Autodesk Inventor part; units mm, degrees
(part 2 of 3)
sketch "스케치16" plane through (0, 0, 0) normal (0, 0, -1) x (-1, 0, 0)
  line L0 (6.921, -57.5) -> (6.921, -59.5) projected
  arc A0 (4.7026, -59.56) -> (6.921, -59.5) centre (5.811, -59.5) ccw projected
  line L1 (4.7026, -59.56) -> (-3.9306, -59.56) projected
  arc A1 (-6.149, -59.5) -> (-3.9306, -59.56) centre (-5.039, -59.5) ccw projected
  line L2 (-6.149, -59.5) -> (-6.149, -57.5) projected
  arc A2 (-3.9306, -57.44) -> (-6.149, -57.5) centre (-5.039, -57.5) ccw projected
  line L3 (-3.9306, -57.44) -> (4.7026, -57.44) projected
  arc A3 (6.921, -57.5) -> (4.7026, -57.44) centre (5.811, -57.5) ccw projected
  line L4 (-14.6916, -62.5) -> (14.3356, -62.5) projected
  arc A4 (14.3356, -62.5) -> (14.361, -62.05) centre (10.361, -62.05) ccw projected
  line L5 (14.361, -62.05) -> (14.361, -54.5339) projected
  arc A5 (14.361, -54.5339) -> (14.2456, -53.5801) centre (10.361, -54.5339) ccw projected
  line L6 (14.2456, -53.5801) -> (5.6489, -18.5692) projected
  arc A6 (5.6489, -18.5692) -> (-6.0049, -18.5692) centre (-0.178, -20) ccw projected
  line L7 (-6.0049, -18.5692) -> (-14.6016, -53.5801) projected
  arc A7 (-14.6016, -53.5801) -> (-14.717, -54.5339) centre (-10.717, -54.5339) ccw projected
  line L8 (-14.717, -54.5339) -> (-14.717, -62.05) projected
  arc A8 (-14.717, -62.05) -> (-14.6916, -62.5) centre (-10.717, -62.05) ccw projected
  circle A9 centre (10.361, -60) radius 1.35 projected
  line L9 (-8.8997, -47.1327) -> (-4.8208, -30.5211) projected
  arc A10 (-0.6725, -27.4837) -> (-4.8208, -30.5211) centre (-0.9362, -31.475) ccw projected
  arc A11 (-0.6725, -27.4837) -> (0.3165, -27.4837) centre (-0.178, -20) ccw projected
  arc A12 (4.4648, -30.5211) -> (0.3165, -27.4837) centre (0.5802, -31.475) ccw projected
  line L10 (4.4648, -30.5211) -> (8.5437, -47.1327) projected
  arc A13 (5.3379, -52.0285) -> (8.5437, -47.1327) centre (4.6591, -48.0865) ccw projected
  arc A14 (-5.694, -52.0285) -> (5.3379, -52.0285) centre (-0.178, -20) ccw projected
  arc A15 (-8.8997, -47.1327) -> (-5.694, -52.0285) centre (-5.0151, -48.0865) ccw projected
  circle A16 centre (-10.639, -60) radius 1.35 projected
  circle A17 centre (-0.178, -20) radius 4 projected
  line L11 (-16.116, -62.5) -> (15.916, -62.5) projected
  arc A18 (15.916, -62.5) -> (16.439, -60.05) centre (10.439, -60.05) ccw projected
  line L12 (16.439, -60.05) -> (16.439, -54.5339) projected
  arc A19 (16.439, -54.5339) -> (16.2659, -53.1031) centre (10.439, -54.5339) ccw projected
  line L13 (16.2659, -53.1031) -> (7.6692, -18.0923) projected
  arc A20 (7.6692, -18.0923) -> (-7.8692, -18.0923) centre (-0.1, -20) ccw projected
  line L14 (-7.8692, -18.0923) -> (-16.4659, -53.1031) projected
  arc A21 (-16.4659, -53.1031) -> (-16.639, -54.5339) centre (-10.639, -54.5339) ccw projected
  line L15 (-16.639, -54.5339) -> (-16.639, -60.05) projected
  arc A22 (-16.639, -60.05) -> (-16.116, -62.5) centre (-10.639, -60.05) ccw projected
  arc A23 (-6.149, -59.5) -> (-3.9306, -59.56) centre (-5.039, -59.5) ccw projected
  line L16 (-6.149, -59.5) -> (-6.149, -57.5) projected
  arc A24 (-3.9306, -57.44) -> (-6.149, -57.5) centre (-5.039, -57.5) ccw projected
  line L17 (-3.9306, -57.44) -> (4.7026, -57.44) projected
  arc A25 (6.921, -57.5) -> (4.7026, -57.44) centre (5.811, -57.5) ccw projected
  line L18 (6.921, -57.5) -> (6.921, -59.5) projected
  arc A26 (4.7026, -59.56) -> (6.921, -59.5) centre (5.811, -59.5) ccw projected
  line L19 (4.7026, -59.56) -> (-3.9306, -59.56) projected
  line L20 (-8.16, -47.3) -> (-8.16, -43.3) projected
  arc A27 (-4.0409, -43.24) -> (-8.16, -43.3) centre (-6.1, -43.3) ccw projected
  line L21 (-4.0409, -43.24) -> (3.8409, -43.24) projected
  arc A28 (7.96, -43.3) -> (3.8409, -43.24) centre (5.9, -43.3) ccw projected
  line L22 (7.96, -43.3) -> (7.96, -47.3) projected
  arc A29 (3.8409, -47.36) -> (7.96, -47.3) centre (5.9, -47.3) ccw projected
  line L23 (3.8409, -47.36) -> (-4.0409, -47.36) projected
  arc A30 (-8.16, -47.3) -> (-4.0409, -47.36) centre (-6.1, -47.3) ccw projected
  line L24 (5.1861, -28.9475) -> (7.0991, -36.7384) projected
  arc A31 (5.7409, -39.1281) -> (7.0991, -36.7384) centre (5.1568, -37.2153) ccw projected
  arc A32 (-5.9409, -39.1281) -> (5.7409, -39.1281) centre (-0.1, -20) ccw projected
  arc A33 (-7.2991, -36.7384) -> (-5.9409, -39.1281) centre (-5.3568, -37.2153) ccw projected
  line L25 (-7.2991, -36.7384) -> (-5.3861, -28.9475) projected
  arc A34 (-2.775, -27.5395) -> (-5.3861, -28.9475) centre (-3.4438, -29.4244) ccw projected
  arc A35 (-2.775, -27.5395) -> (2.575, -27.5395) centre (-0.1, -20) ccw projected
  arc A36 (5.1861, -28.9475) -> (2.575, -27.5395) centre (3.2438, -29.4244) ccw projected
  circle A37 centre (-11.1, -45.3) radius 1.35 projected
  circle A38 centre (10.9, -45.3) radius 1.35 projected
  circle A39 centre (-0.1, -20) radius 4 projected
  circle A40 centre (-10.639, -60) radius 1.35 projected
  circle A41 centre (10.361, -60) radius 1.35 projected
  line L26 (-15.5728, -53.3416) -> (-6.9761, -18.3308)
  arc A42 (6.62, -18.3308) -> (-6.9761, -18.3308) centre (-0.178, -20) ccw
  line L27 (6.62, -18.3308) -> (15.2167, -53.3416)
  arc A43 (15.361, -54.5339) -> (15.2167, -53.3416) centre (10.361, -54.5339) ccw
  line L28 (15.361, -54.5339) -> (15.361, -62.05)
  arc A44 (15.1461, -63.5) -> (15.361, -62.05) centre (10.361, -62.05) ccw
  line L29 (15.1461, -63.5) -> (-15.5022, -63.5)
  arc A45 (-15.717, -62.05) -> (-15.5022, -63.5) centre (-10.717, -62.05) ccw
  line L30 (-15.717, -62.05) -> (-15.717, -54.5339)
  arc A46 (-15.5728, -53.3416) -> (-15.717, -54.5339) centre (-10.717, -54.5339) ccw
  point P0 (0, 0)
  point P1 (-15.6967, -62.5)
  point P2 (15.3407, -62.5)
  dimension "d62" = 1
  constraints: 10 end point, 10 point on circle, 5 centre point, 9 other
  measures "d62" distance between parallel lines of L7 L26
extrude "돌출16" cut sketch "스케치16" against normal through all contours L11 A22 L15 A21 L14 A20 L13 A19 L12 A18 A44 L28 A43 L27 A42 L26 A46 L30 A45
sketch "스케치17" plane through (0, 0, 0) normal (0, 0, -1) x (-1, 0, 0)
  circle A0 centre (10.361, -60) radius 1.35 projected
  circle A1 centre (-10.639, -60) radius 1.35 projected
  circle A2 centre (-0.1, -20) radius 4 projected
  circle A3 centre (10.9, -45.3) radius 1.35 projected
  circle A4 centre (-11.1, -45.3) radius 1.35 projected
  line L0 (5.1861, -28.9475) -> (7.0991, -36.7384) projected
  arc A5 (5.7409, -39.1281) -> (7.0991, -36.7384) centre (5.1568, -37.2153) ccw projected
  arc A6 (-5.9409, -39.1281) -> (5.7409, -39.1281) centre (-0.1, -20) ccw projected
  arc A7 (-7.2991, -36.7384) -> (-5.9409, -39.1281) centre (-5.3568, -37.2153) ccw projected
  line L1 (-7.2991, -36.7384) -> (-5.3861, -28.9475) projected
  arc A8 (-2.775, -27.5395) -> (-5.3861, -28.9475) centre (-3.4438, -29.4244) ccw projected
  arc A9 (-2.775, -27.5395) -> (2.575, -27.5395) centre (-0.1, -20) ccw projected
  arc A10 (5.1861, -28.9475) -> (2.575, -27.5395) centre (3.2438, -29.4244) ccw projected
  line L2 (-8.16, -47.3) -> (-8.16, -43.3) projected
  arc A11 (-4.0409, -43.24) -> (-8.16, -43.3) centre (-6.1, -43.3) ccw projected
  line L3 (-4.0409, -43.24) -> (3.8409, -43.24) projected
  arc A12 (7.96, -43.3) -> (3.8409, -43.24) centre (5.9, -43.3) ccw projected
  line L4 (7.96, -43.3) -> (7.96, -47.3) projected
  arc A13 (3.8409, -47.36) -> (7.96, -47.3) centre (5.9, -47.3) ccw projected
  line L5 (3.8409, -47.36) -> (-4.0409, -47.36) projected
  arc A14 (-8.16, -47.3) -> (-4.0409, -47.36) centre (-6.1, -47.3) ccw projected
  arc A15 (-6.149, -59.5) -> (-3.9306, -59.56) centre (-5.039, -59.5) ccw projected
  line L6 (-6.149, -59.5) -> (-6.149, -57.5) projected
  arc A16 (-3.9306, -57.44) -> (-6.149, -57.5) centre (-5.039, -57.5) ccw projected
  line L7 (-3.9306, -57.44) -> (4.7026, -57.44) projected
  arc A17 (6.921, -57.5) -> (4.7026, -57.44) centre (5.811, -57.5) ccw projected
  line L8 (6.921, -57.5) -> (6.921, -59.5) projected
  arc A18 (4.7026, -59.56) -> (6.921, -59.5) centre (5.811, -59.5) ccw projected
  line L9 (4.7026, -59.56) -> (-3.9306, -59.56) projected
  arc A19 (15.3407, -62.5) -> (15.361, -62.05) centre (10.361, -62.05) ccw projected
  line L10 (15.361, -62.05) -> (15.361, -54.5339) projected
  arc A20 (15.361, -54.5339) -> (15.2167, -53.3416) centre (10.361, -54.5339) ccw projected
  line L11 (15.2167, -53.3416) -> (6.62, -18.3308) projected
  arc A21 (6.62, -18.3308) -> (-6.9761, -18.3308) centre (-0.178, -20) ccw projected
  line L12 (-6.9761, -18.3308) -> (-15.5728, -53.3416) projected
  arc A22 (-15.5728, -53.3416) -> (-15.717, -54.5339) centre (-10.717, -54.5339) ccw projected
  line L13 (-15.717, -54.5339) -> (-15.717, -62.05) projected
  arc A23 (-15.717, -62.05) -> (-15.6967, -62.5) centre (-10.717, -62.05) ccw projected
  line L14 (-15.6967, -62.5) -> (15.3407, -62.5) projected
  line L15 (15.361, -54.5339) -> (-15.717, -54.5339)
  line L16 (-15.717, -54.5339) -> (-15.717, -62.5)
  line L17 (-15.717, -62.5) -> (15.361, -62.5)
  line L18 (15.361, -62.5) -> (15.361, -54.5339)
  point P0 (0, 0)
  point P1 (15.361, -62.05)
  point P2 (15.3407, -62.5)
  constraints: 8 end point, 2 parallel, 1 horizontal, 1 perpendicular
extrude "돌출17" add sketch "스케치17" against normal blind 2 contours A19 L18 L17 | L17 L16 A23
sketch "스케치18" plane through (0, 0, 2) normal (0, 0, 1) x (1, 0, 0)
  line L0 (-15.361, -62.5) -> (15.717, -62.5) projected
  line L1 (15.717, -62.5) -> (15.717, -54.5339) projected
  arc A0 (15.717, -54.5339) -> (15.5728, -53.3416) centre (10.717, -54.5339) ccw projected
  line L2 (15.5728, -53.3416) -> (6.9761, -18.3308) projected
  arc A1 (6.9761, -18.3308) -> (-6.62, -18.3308) centre (0.178, -20) ccw projected
  line L3 (-6.62, -18.3308) -> (-15.2167, -53.3416) projected
  arc A2 (-15.2167, -53.3416) -> (-15.361, -54.5339) centre (-10.361, -54.5339) ccw projected
  line L4 (-15.361, -54.5339) -> (-15.361, -62.5) projected
  line L5 (8.16, -43.3) -> (8.16, -47.3) projected
  arc A3 (4.0409, -47.36) -> (8.16, -47.3) centre (6.1, -47.3) ccw projected
  line L6 (4.0409, -47.36) -> (-3.8409, -47.36) projected
  arc A4 (-7.96, -47.3) -> (-3.8409, -47.36) centre (-5.9, -47.3) ccw projected
  line L7 (-7.96, -47.3) -> (-7.96, -43.3) projected
  arc A5 (-3.8409, -43.24) -> (-7.96, -43.3) centre (-5.9, -43.3) ccw projected
  line L8 (-3.8409, -43.24) -> (4.0409, -43.24) projected
  arc A6 (8.16, -43.3) -> (4.0409, -43.24) centre (6.1, -43.3) ccw projected
  line L9 (-7.0991, -36.7384) -> (-5.1861, -28.9475) projected
  arc A7 (-2.575, -27.5395) -> (-5.1861, -28.9475) centre (-3.2438, -29.4244) ccw projected
  arc A8 (-2.575, -27.5395) -> (2.775, -27.5395) centre (0.1, -20) ccw projected
  arc A9 (5.3861, -28.9475) -> (2.775, -27.5395) centre (3.4438, -29.4244) ccw projected
  line L10 (5.3861, -28.9475) -> (7.2991, -36.7384) projected
  arc A10 (5.9409, -39.1281) -> (7.2991, -36.7384) centre (5.3568, -37.2153) ccw projected
  arc A11 (-5.7409, -39.1281) -> (5.9409, -39.1281) centre (0.1, -20) ccw projected
  arc A12 (-7.0991, -36.7384) -> (-5.7409, -39.1281) centre (-5.1568, -37.2153) ccw projected
  circle A13 centre (11.1, -45.3) radius 1.35 projected
  circle A14 centre (-10.9, -45.3) radius 1.35 projected
  circle A15 centre (10.639, -60) radius 1.35 projected
  circle A16 centre (-10.361, -60) radius 1.35 projected
  circle A17 centre (0.1, -20) radius 4 projected
  arc A18 (3.9306, -59.56) -> (6.149, -59.5) centre (5.039, -59.5) ccw projected
  line L11 (3.9306, -59.56) -> (-4.7026, -59.56) projected
  arc A19 (-6.921, -59.5) -> (-4.7026, -59.56) centre (-5.811, -59.5) ccw projected
  line L12 (-6.921, -59.5) -> (-6.921, -57.5) projected
  arc A20 (-4.7026, -57.44) -> (-6.921, -57.5) centre (-5.811, -57.5) ccw projected
  line L13 (-4.7026, -57.44) -> (3.9306, -57.44) projected
  arc A21 (6.149, -57.5) -> (3.9306, -57.44) centre (5.039, -57.5) ccw projected
  line L14 (6.149, -57.5) -> (6.149, -59.5) projected
  point P0 (0, 0)
extrude "돌출18" add sketch "스케치18" against normal blind 2 contours L5 A3 L6 A4 L7 A5 L8 A6 | A13 | A14 | L11 A19 L12 A20 L13 A21 L14 A18
sketch "스케치19" plane through (0, 0, 2) normal (0, 0, 1) x (1, 0, 0)
  line L0 (-15.361, -62.5) -> (15.717, -62.5) projected
  line L1 (15.717, -62.5) -> (15.717, -54.5339) projected
  arc A0 (15.717, -54.5339) -> (15.5728, -53.3416) centre (10.717, -54.5339) ccw projected
  line L2 (15.5728, -53.3416) -> (6.9761, -18.3308) projected
  arc A1 (6.9761, -18.3308) -> (-6.62, -18.3308) centre (0.178, -20) ccw projected
  line L3 (-6.62, -18.3308) -> (-15.2167, -53.3416) projected
  arc A2 (-15.2167, -53.3416) -> (-15.361, -54.5339) centre (-10.361, -54.5339) ccw projected
  line L4 (-15.361, -54.5339) -> (-15.361, -62.5) projected
  line L5 (-7.0991, -36.7384) -> (-5.1861, -28.9475) projected
  arc A3 (-2.575, -27.5395) -> (-5.1861, -28.9475) centre (-3.2438, -29.4244) ccw projected
  arc A4 (-2.575, -27.5395) -> (2.775, -27.5395) centre (0.1, -20) ccw projected
  arc A5 (5.3861, -28.9475) -> (2.775, -27.5395) centre (3.4438, -29.4244) ccw projected
  line L6 (5.3861, -28.9475) -> (7.2991, -36.7384) projected
  arc A6 (5.9409, -39.1281) -> (7.2991, -36.7384) centre (5.3568, -37.2153) ccw projected
  arc A7 (-5.7409, -39.1281) -> (5.9409, -39.1281) centre (0.1, -20) ccw projected
  arc A8 (-7.0991, -36.7384) -> (-5.7409, -39.1281) centre (-5.1568, -37.2153) ccw projected
  circle A9 centre (10.639, -60) radius 1.35 projected
  circle A10 centre (-10.361, -60) radius 1.35 projected
  circle A11 centre (0.1, -20) radius 4 projected
  line L7 (7.199, -57.5) -> (7.199, -59.5) projected
  arc A12 (4.9806, -59.56) -> (7.199, -59.5) centre (6.089, -59.5) ccw projected
  line L8 (4.9806, -59.56) -> (-3.6526, -59.56) projected
  arc A13 (-5.871, -59.5) -> (-3.6526, -59.56) centre (-4.761, -59.5) ccw projected
  line L9 (-5.871, -59.5) -> (-5.871, -57.5) projected
  arc A14 (-3.6526, -57.44) -> (-5.871, -57.5) centre (-4.761, -57.5) ccw projected
  line L10 (-3.6526, -57.44) -> (4.9806, -57.44) projected
  arc A15 (7.199, -57.5) -> (4.9806, -57.44) centre (6.089, -57.5) ccw projected
  line L11 (-14.4136, -62.5) -> (14.6136, -62.5) projected
  arc A16 (14.6136, -62.5) -> (14.639, -62.05) centre (10.639, -62.05) ccw projected
  line L12 (14.639, -62.05) -> (14.639, -54.5339) projected
  arc A17 (14.639, -54.5339) -> (14.5236, -53.5801) centre (10.639, -54.5339) ccw projected
  line L13 (14.5236, -53.5801) -> (5.9269, -18.5692) projected
  arc A18 (5.9269, -18.5692) -> (-5.7269, -18.5692) centre (0.1, -20) ccw projected
  line L14 (-5.7269, -18.5692) -> (-14.3236, -53.5801) projected
  arc A19 (-14.3236, -53.5801) -> (-14.439, -54.5339) centre (-10.439, -54.5339) ccw projected
  line L15 (-14.439, -54.5339) -> (-14.439, -62.05) projected
  arc A20 (-14.439, -62.05) -> (-14.4136, -62.5) centre (-10.439, -62.05) ccw projected
  circle A21 centre (10.639, -60) radius 1.35 projected
  line L16 (-8.6217, -47.1327) -> (-4.5428, -30.5211) projected
  arc A22 (-0.3945, -27.4837) -> (-4.5428, -30.5211) centre (-0.6582, -31.475) ccw projected
  arc A23 (-0.3945, -27.4837) -> (0.5945, -27.4837) centre (0.1, -20) ccw projected
  arc A24 (4.7428, -30.5211) -> (0.5945, -27.4837) centre (0.8582, -31.475) ccw projected
  line L17 (4.7428, -30.5211) -> (8.8217, -47.1327) projected
  arc A25 (5.616, -52.0285) -> (8.8217, -47.1327) centre (4.9371, -48.0865) ccw projected
  arc A26 (-5.416, -52.0285) -> (5.616, -52.0285) centre (0.1, -20) ccw projected
  arc A27 (-8.6217, -47.1327) -> (-5.416, -52.0285) centre (-4.7371, -48.0865) ccw projected
  circle A28 centre (-10.361, -60) radius 1.35 projected
  circle A29 centre (0.1, -20) radius 4 projected
  arc A30 (20.1, 4.5766) -> (19.5808, 6.2636) centre (17.1, 4.5766) ccw projected
  line L18 (19.5808, 6.2636) -> (15.5953, 12.1246) projected
  arc A31 (15.5953, 12.1246) -> (13.9414, 13) centre (13.9414, 11) ccw projected
  line L19 (13, 13) -> (13.9414, 13) projected
  arc A32 (14.5, 11.5) -> (13, 13) centre (13, 11.5) ccw projected
  line L20 (14.5, -41.5) -> (14.5, 11.5) projected
  arc A33 (13.5, -42.5) -> (14.5, -41.5) centre (13.5, -41.5) ccw projected
  line L21 (-13.5, -42.5) -> (13.5, -42.5) projected
  arc A34 (-14.5, -41.5) -> (-13.5, -42.5) centre (-13.5, -41.5) ccw projected
  line L22 (-14.5, 11.5) -> (-14.5, -41.5) projected
  arc A35 (-13, 13) -> (-14.5, 11.5) centre (-13, 11.5) ccw projected
  line L23 (-13.9414, 13) -> (-13, 13) projected
  arc A36 (-13.9414, 13) -> (-15.5953, 12.1246) centre (-13.9414, 11) ccw projected
  line L24 (-15.5953, 12.1246) -> (-19.5808, 6.2636) projected
  arc A37 (-19.5808, 6.2636) -> (-20.1, 4.5766) centre (-17.1, 4.5766) ccw projected
  line L25 (-20.1, 4.5766) -> (-20.1, -39.6766) projected
  arc A38 (-20.1, -39.6766) -> (-19.5808, -41.3636) centre (-17.1, -39.6766) ccw projected
  line L26 (-19.5808, -41.3636) -> (-15.8929, -46.7869) projected
  arc A39 (-15.8929, -46.7869) -> (-13.4121, -48.1) centre (-13.4121, -45.1) ccw projected
  line L27 (-13.4121, -48.1) -> (13.4121, -48.1) projected
  arc A40 (13.4121, -48.1) -> (15.8929, -46.7869) centre (13.4121, -45.1) ccw projected
  line L28 (15.8929, -46.7869) -> (19.5808, -41.3636) projected
  arc A41 (19.5808, -41.3636) -> (20.1, -39.6766) centre (17.1, -39.6766) ccw projected
  line L29 (20.1, -39.6766) -> (20.1, 4.5766) projected
  circle A42 centre (-17.3, 4) radius 1.35 projected
  circle A43 centre (-17.3, -18) radius 1.35 projected
  circle A44 centre (-11, -45.3) radius 1.35 projected
  circle A45 centre (17.3, 4) radius 1.35 projected
  circle A46 centre (17.3, -18) radius 1.35 projected
  circle A47 centre (11, -45.3) radius 1.35 projected
  circle A48 centre (-17.3, -40) radius 1.35 projected
  circle A49 centre (17.3, -40) radius 1.35 projected
  point P0 (0, 0)
extrude "돌출19" cut sketch "스케치19" against normal blind 2 contours A44 L14 | L14 A44 | L7 A12 L8 A13 L9 A14 L10 A15 | A47
sketch "스케치20" plane through (0, 0, 2) normal (0, 0, 1) x (1, 0, 0)
  circle A0 centre (-4.4, -45.3) radius 1 projected
  circle A1 centre (4.4, -45.3) radius 1 projected
  line L0 (8, -43.3) -> (8, -47.3) projected
  line L1 (-8, -43.3) -> (8, -43.3) projected
  line L2 (-8, -47.3) -> (-8, -43.3) projected
  line L3 (8, -47.3) -> (-8, -47.3) projected
  line L4 (-8.06, -47.36) -> (-8.06, -43.24)
  line L5 (-8.06, -43.24) -> (8.06, -43.24)
  line L6 (8.06, -43.24) -> (8.06, -47.36)
  line L7 (8.06, -47.36) -> (-8.06, -47.36)
  line L8 (8.06, -47.36) -> (8.06, -43.24)
  line L9 (-22.2818, -39.9612) -> (-22.2818, -44.0812)
  line L10 (-22.2818, -44.0812) -> (-22.2818, -39.9612) construction
  line L11 (-20.7818, -44.0812) -> (-20.7818, -39.9612)
  line L12 (-23.7818, -39.9612) -> (-23.7818, -44.0812)
  arc A2 (-23.7818, -44.0812) -> (-20.7818, -44.0812) centre (-22.2818, -44.0812) ccw
  arc A3 (-20.7818, -39.9612) -> (-23.7818, -39.9612) centre (-22.2818, -39.9612) ccw
  line L13 (6.56, -43.24) -> (6.56, -47.36)
  line L14 (6.56, -47.36) -> (6.56, -43.24) construction
  line L15 (8.06, -47.36) -> (8.06, -43.24)
  line L16 (5.06, -43.24) -> (5.06, -47.36)
  arc A4 (5.06, -47.36) -> (8.06, -47.36) centre (6.56, -47.36) ccw
  arc A5 (8.06, -43.24) -> (5.06, -43.24) centre (6.56, -43.24) ccw
  line L17 (-6.56, -43.24) -> (-6.56, -47.36)
  line L18 (-6.56, -47.36) -> (-6.56, -43.24) construction
  line L19 (-5.06, -47.36) -> (-5.06, -43.24)
  line L20 (-8.06, -43.24) -> (-8.06, -47.36)
  arc A6 (-8.06, -47.36) -> (-5.06, -47.36) centre (-6.56, -47.36) ccw
  arc A7 (-5.06, -43.24) -> (-8.06, -43.24) centre (-6.56, -43.24) ccw
  point P0 (0, 0)
  point P1 (-22.2818, -42.0212)
  point P2 (6.56, -45.3)
  point P3 (-6.56, -45.3)
  point P4 (5.06, -43.3)
  point P5 (-5.06, -43.3)
  dimension "d71" = 0.06
  dimension "d72" = 3
  dimension "d73" = 3
  dimension "d74" = 3
  constraints: 40 end point, 12 point on circle, 12 tangent, 6 centre point, 4 vertical, 3 midpoint, 3 parallel, 3 other
  measures "d71" distance between parallel lines of L3 L7
  measures "d72" diameter of A3
  measures "d73" diameter of A5
  measures "d74" diameter of A7
extrude "돌출20" cut sketch "스케치20" against normal blind 2 contours A0 L19 | A0 L19 L1 L16 A1 L3 | L19 A0 | A0 L19 L3 L17 L1 | L1 L17 L5 L19 | L19 L7 L17 L3 | L3 L16 L7 L19 | L17 L3 L2 L1 | L1 L2 L3 L17 L7 L4 L5 | L16 L5 L13 L1 | L1 L13 L3 L16 A1 | L5 A7 | L3 L13 L7 L16 | A6 L7 | L13 L5 L6 L7 L3 L0 L1 | L1 L0 L3 L13 | A5 L5 | L16 A1 | A1 L16 | L7 A4
sketch "스케치21" plane through (0, 0, 0) normal (0, 0, -1) x (-1, 0, 0)
  arc A0 (8.06, -43.24) -> (5.06, -43.24) centre (6.56, -43.24) ccw projected
  line L0 (8.06, -43.24) -> (8.06, -47.36) projected
  arc A1 (5.06, -47.36) -> (8.06, -47.36) centre (6.56, -47.36) ccw projected
  line L1 (5.06, -47.36) -> (-5.06, -47.36) projected
  arc A2 (-8.06, -47.36) -> (-5.06, -47.36) centre (-6.56, -47.36) ccw projected
  line L2 (-8.06, -47.36) -> (-8.06, -43.24) projected
  arc A3 (-5.06, -43.24) -> (-8.06, -43.24) centre (-6.56, -43.24) ccw projected
  line L3 (-5.06, -43.24) -> (-5.06, -43.3) projected
  line L4 (-5.06, -43.3) -> (5.06, -43.3) projected
  line L5 (5.06, -43.3) -> (5.06, -43.24) projected
  circle A4 centre (-11, -45.3) radius 1.35 projected
  circle A5 centre (11, -45.3) radius 1.35 projected
  arc A6 (3.6526, -59.56) -> (5.871, -59.5) centre (4.761, -59.5) ccw projected
  line L6 (3.6526, -59.56) -> (-4.9806, -59.56) projected
  arc A7 (-7.199, -59.5) -> (-4.9806, -59.56) centre (-6.089, -59.5) ccw projected
  line L7 (-7.199, -59.5) -> (-7.199, -57.5) projected
  arc A8 (-4.9806, -57.44) -> (-7.199, -57.5) centre (-6.089, -57.5) ccw projected
  line L8 (-4.9806, -57.44) -> (3.6526, -57.44) projected
  arc A9 (5.871, -57.5) -> (3.6526, -57.44) centre (4.761, -57.5) ccw projected
  line L9 (5.871, -57.5) -> (5.871, -59.5) projected
  circle A10 centre (10.361, -60) radius 1.35 projected
  circle A11 centre (-10.639, -60) radius 1.35 projected
  circle A12 centre (-0.1, -20) radius 4 projected
  line L10 (5.1861, -28.9475) -> (7.0991, -36.7384) projected
  arc A13 (5.7409, -39.1281) -> (7.0991, -36.7384) centre (5.1568, -37.2153) ccw projected
  arc A14 (-5.9409, -39.1281) -> (5.7409, -39.1281) centre (-0.1, -20) ccw projected
  arc A15 (-7.2991, -36.7384) -> (-5.9409, -39.1281) centre (-5.3568, -37.2153) ccw projected
  line L11 (-7.2991, -36.7384) -> (-5.3861, -28.9475) projected
  arc A16 (-2.775, -27.5395) -> (-5.3861, -28.9475) centre (-3.4438, -29.4244) ccw projected
  arc A17 (-2.775, -27.5395) -> (2.575, -27.5395) centre (-0.1, -20) ccw projected
  arc A18 (5.1861, -28.9475) -> (2.575, -27.5395) centre (3.2438, -29.4244) ccw projected
  line L12 (15.361, -62.5) -> (15.361, -54.5339) projected
  arc A19 (15.361, -54.5339) -> (15.2167, -53.3416) centre (10.361, -54.5339) ccw projected
  line L13 (15.2167, -53.3416) -> (6.62, -18.3308) projected
  arc A20 (6.62, -18.3308) -> (-6.9761, -18.3308) centre (-0.178, -20) ccw projected
  line L14 (-6.9761, -18.3308) -> (-15.5728, -53.3416) projected
  arc A21 (-15.5728, -53.3416) -> (-15.717, -54.5339) centre (-10.717, -54.5339) ccw projected
  line L15 (-15.717, -54.5339) -> (-15.717, -62.5) projected
  line L16 (-15.717, -62.5) -> (15.361, -62.5) projected
  point P0 (0, 0)
  point P1 (-13.6725, -37.0927)
  constraints: 1 other
extrude "돌출21" add sketch "스케치21" against normal blind 2 contours L0 A1 L1 A2 L2 A3 L3 L4 L5 A0 | A4 | A5 | L6 A7 L7 A8 L8 A9 L9 A6 | A10 | A11
sketch "스케치22" plane through (0, 0, 0) normal (0, 0, -1) x (-1, 0, 0)
  line L0 (7.3148, -57.5317) -> (7.3064, -59.5317) projected
  arc A0 (5.1878, -59.5827) -> (7.3064, -59.5317) centre (6.2464, -59.5272) ccw projected
  line L1 (5.1878, -59.5827) -> (-5.7227, -59.5366) projected
  arc A1 (-7.8407, -59.4676) -> (-5.7227, -59.5366) centre (-6.7807, -59.4721) ccw projected
  line L2 (-7.8407, -59.4676) -> (-7.8323, -57.4676) projected
  arc A2 (-5.7137, -57.4166) -> (-7.8323, -57.4676) centre (-6.7723, -57.4721) ccw projected
  line L3 (-5.7137, -57.4166) -> (5.1968, -57.4628) projected
  arc A3 (7.3148, -57.5317) -> (5.1968, -57.4628) centre (6.2548, -57.5272) ccw projected
  circle A4 centre (-12.2828, -59.9488) radius 1.35 projected
  circle A5 centre (11.7442, -60.0505) radius 1.35 projected
  line L4 (-14.8188, -62.4381) -> (14.259, -62.5612) projected
  line L5 (14.259, -62.5612) -> (14.2927, -54.5951) projected
  arc A6 (14.2927, -54.5951) -> (14.1814, -53.6408) centre (10.2927, -54.5782) ccw projected
  line L6 (14.1814, -53.6408) -> (5.7329, -18.5939) projected
  arc A7 (5.7329, -18.5939) -> (-5.9208, -18.5446) centre (-0.1, -20) ccw projected
  line L7 (-5.9208, -18.5446) -> (-14.6656, -53.5187) projected
  arc A8 (-14.6656, -53.5187) -> (-14.7851, -54.4721) centre (-10.7851, -54.489) ccw projected
  line L8 (-14.7851, -54.4721) -> (-14.8188, -62.4381) projected
  line L9 (-8.9364, -47.0955) -> (-4.7873, -30.5014) projected
  arc A9 (-0.6262, -27.4815) -> (-4.7873, -30.5014) centre (-0.9068, -31.4717) ccw projected
  arc A10 (-0.6262, -27.4815) -> (0.3628, -27.4857) centre (-0.1, -20) ccw projected
  arc A11 (4.4982, -30.5407) -> (0.3628, -27.4857) centre (0.6096, -31.4781) ccw projected
  line L10 (4.4982, -30.5407) -> (8.5068, -47.1694) projected
  arc A12 (5.2803, -52.0515) -> (8.5068, -47.1694) centre (4.6182, -48.1067) ccw projected
  arc A13 (-5.7515, -52.0049) -> (5.2803, -52.0515) centre (-0.1, -20) ccw projected
  arc A14 (-8.9364, -47.0955) -> (-5.7515, -52.0049) centre (-5.0559, -48.0658) ccw projected
  circle A15 centre (-0.1, -20) radius 4 projected
  point P0 (0, 0)
extrude "돌출22" cut sketch "스케치22" against normal blind 2 contours L0 A0 L1 A1 L2 A2 L3 A3 | A4 | A5
sketch "스케치23" plane through (0, 0, 2) normal (0, 0, 1) x (1, 0, 0)
  circle A0 centre (4.607, -45.2811) radius 1 projected
  circle A1 centre (-4.1929, -45.3184) radius 1 projected
  line L0 (-7.8013, -43.3337) -> (-7.7844, -47.3336) projected
  line L1 (8.1985, -43.2659) -> (-7.8013, -43.3337) projected
  line L2 (8.2155, -47.2659) -> (8.1985, -43.2659) projected
  line L3 (-7.7844, -47.3336) -> (8.2155, -47.2659) projected
  circle A2 centre (-10.7928, -45.3463) radius 1 projected
  line L4 (-8.9013, -43.3383) -> (-8.8844, -47.3383) projected
  line L5 (-8.8844, -47.3383) -> (-12.7843, -47.3548) projected
  line L6 (-12.7843, -47.3548) -> (-12.8013, -43.3548) projected
  line L7 (-12.8013, -43.3548) -> (-8.9013, -43.3383) projected
  circle A3 centre (11.207, -45.2532) radius 1 projected
  line L8 (9.3155, -47.2612) -> (9.2985, -43.2613) projected
  line L9 (9.2985, -43.2613) -> (13.1985, -43.2448) projected
  line L10 (13.1985, -43.2448) -> (13.2154, -47.2447) projected
  line L11 (13.2154, -47.2447) -> (9.3155, -47.2612) projected
  circle A4 centre (11.207, -45.2532) radius 1.35
  circle A5 centre (-10.7928, -45.3463) radius 1.35
  line L12 (0.2156, -47.2998) -> (0.1986, -43.2998)
  line L13 (0.2156, -47.2998) -> (0.1986, -43.2998) construction
  line L14 (1.2155, -47.2955) -> (1.1986, -43.2956)
  line L15 (-0.8014, -43.304) -> (-0.7844, -47.304)
  arc A6 (-0.7844, -47.304) -> (1.2155, -47.2955) centre (0.2156, -47.2998) ccw
  arc A7 (1.1986, -43.2956) -> (-0.8014, -43.304) centre (0.1986, -43.2998) ccw
  line L16 (8.2155, -47.2659) -> (8.1985, -43.2659)
  line L17 (8.1985, -43.2659) -> (7.1986, -43.2702)
  line L18 (7.1986, -43.2702) -> (7.2155, -47.2701)
  line L19 (7.2155, -47.2701) -> (8.2155, -47.2659)
  line L20 (-7.7844, -47.3336) -> (-7.8013, -43.3337)
  line L21 (-7.8013, -43.3337) -> (-6.8013, -43.3294)
  line L22 (-6.8013, -43.3294) -> (-6.7844, -47.3294)
  line L23 (-6.7844, -47.3294) -> (-7.7844, -47.3336)
  line L24 (7.2155, -47.2998) -> (7.1986, -43.2998)
  line L25 (7.2155, -47.2998) -> (7.1986, -43.2998) construction
  line L26 (8.2155, -47.2955) -> (8.1985, -43.2956)
  line L27 (6.1986, -43.304) -> (6.2155, -47.304)
  arc A8 (6.2155, -47.304) -> (8.2155, -47.2955) centre (7.2155, -47.2998) ccw
  arc A9 (8.1985, -43.2956) -> (6.1986, -43.304) centre (7.1986, -43.2998) ccw
  line L28 (-6.7844, -47.3294) -> (-6.8013, -43.3294)
  line L29 (-6.7844, -47.3294) -> (-6.8013, -43.3294) construction
  line L30 (-5.7844, -47.3252) -> (-5.8013, -43.3252)
  line L31 (-7.8013, -43.3337) -> (-7.7844, -47.3336)
  arc A10 (-7.7844, -47.3336) -> (-5.7844, -47.3252) centre (-6.7844, -47.3294) ccw
  arc A11 (-5.8013, -43.3252) -> (-7.8013, -43.3337) centre (-6.8013, -43.3294) ccw
  line L32 (8.2757, -47.3256) -> (8.2583, -43.2057)
  line L33 (8.2583, -43.2057) -> (-7.8616, -43.2739)
  line L34 (-7.8616, -43.2739) -> (-7.8441, -47.3939)
  line L35 (-7.8441, -47.3939) -> (8.2757, -47.3256)
  line L36 (8.2755, -47.2953) -> (8.2585, -43.2953)
  arc A12 (8.2585, -43.2953) -> (6.1386, -43.3043) centre (7.1986, -43.2998) ccw
  line L37 (6.1386, -43.3043) -> (6.1555, -47.3042)
  arc A13 (6.1555, -47.3042) -> (8.2755, -47.2953) centre (7.2155, -47.2998) ccw
  line L38 (-5.7244, -47.3249) -> (-5.7413, -43.3249)
  arc A14 (-5.7413, -43.3249) -> (-7.8613, -43.3339) centre (-6.8013, -43.3294) ccw
  line L39 (-7.8613, -43.3339) -> (-7.8444, -47.3339)
  arc A15 (-7.8444, -47.3339) -> (-5.7244, -47.3249) centre (-6.7844, -47.3294) ccw
  point P0 (0, 0)
  point P1 (0.2071, -45.2998)
  point P2 (7.207, -45.2998)
  point P3 (-6.7929, -45.3294)
  point P4 (6.1989, -43.2744)
  point P5 (6.2154, -47.2744)
  point P6 (-7.8424, -47.3939)
  point P7 (-5.7258, -47.3849)
  point P8 (6.1561, -47.3346)
  point P9 (8.2752, -47.3256)
  point P10 (8.2544, -43.2057)
  point P11 (6.142, -43.2146)
  point P12 (-5.7433, -43.2649)
  point P13 (-7.8599, -43.2739)
  dimension "d81" = 2.7
  dimension "d82" = 2.7
  dimension "d83" = 2
  dimension "d84" = 1
  dimension "d85" = 1
  dimension "d86" = 2
  dimension "d87" = 2
  dimension "d90" = 0.06
  dimension "d91" = 0.06
  dimension "d92" = 0.06
  constraints: 62 end point, 20 point on circle, 13 equal length, 12 centre point, 12 tangent, 5 midpoint, 2 coincident, 2 perpendicular, 9 other
  measures "d81" diameter of A4
  measures "d82" diameter of A5
  measures "d83" diameter of A7
  measures "d84" distance of L17.end L1.start
  measures "d85" distance of L0.start L21.end
  measures "d86" diameter of A9
  measures "d87" diameter of A11
  measures "d90" distance between parallel lines of L3 L35
  measures "d91" radial gap between concentric circles of A8 A13
  measures "d92" radial gap between concentric circles of A10 A15
extrude "돌출23" cut sketch "스케치23" against normal blind 2 contours A0 | A1 | L1 L22 L3 L0 | A11 L33 L1 | L0 A10 L35 L34 L33 A11 | L3 A10 L35 | L1 L30 L3 L22 | L33 A14 A11 | A11 L33 | L35 A10 | A10 L35 A15 | A11 L33 A14 L1 | L1 L38 L3 L30 | L3 A15 L35 A10 | A14 L33 A7 L1 | L1 L15 L3 L38 | L3 A6 L35 A15 | A7 L33 L1 | L1 L12 L3 L15 | L3 A6 L35 | L1 L14 L3 L12 | L33 A12 L1 A7 | A6 L3 L37 A13 L35 | L1 A12 L37 L3 L14 | A12 L33 A9 | L33 A9 L1 A12 | A13 L37 L3 L27 A8 L35 | L35 A8 A13 | L1 A9 L27 L3 L37 A12 | L33 A9 L1 | A9 L33 | A12 L32 L35 A8 L26 L2 A9 L33 | L33 L32 A12 | L35 A8 | A8 L27 L3 L26 L35 | L1 L18 L3 L27 A9 | L1 L2 L3 L18 | A2 | A3 | A4 | A5
sketch "스케치24" plane through (0, 0, 0) normal (0, 0, -1) x (-1, 0, 0)
  circle A0 centre (10.7928, -45.3463) radius 1.35 projected
  circle A1 centre (-11.207, -45.2532) radius 1.35 projected
  arc A2 (-8.2752, -47.3256) -> (-6.1561, -47.3346) centre (-7.2155, -47.2998) ccw projected
  line L0 (-8.2752, -47.3256) -> (-8.2757, -47.3256) projected
  line L1 (-8.2757, -47.3256) -> (-8.2583, -43.2057) projected
  line L2 (-8.2583, -43.2057) -> (-8.2544, -43.2057) projected
  arc A3 (-6.142, -43.2146) -> (-8.2544, -43.2057) centre (-7.1986, -43.2998) ccw projected
  line L3 (-6.142, -43.2146) -> (5.7433, -43.2649) projected
  arc A4 (7.8599, -43.2739) -> (5.7433, -43.2649) centre (6.8013, -43.3294) ccw projected
  line L4 (7.8599, -43.2739) -> (7.8616, -43.2739) projected
  line L5 (7.8616, -43.2739) -> (7.8441, -47.3939) projected
  line L6 (7.8441, -47.3939) -> (7.8424, -47.3939) projected
  arc A5 (5.7258, -47.3849) -> (7.8424, -47.3939) centre (6.7844, -47.3294) ccw projected
  line L7 (5.7258, -47.3849) -> (-6.1561, -47.3346) projected
  circle A6 centre (-12.2828, -59.9488) radius 1.35 projected
  arc A7 (-7.8407, -59.4676) -> (-5.7227, -59.5366) centre (-6.7807, -59.4721) ccw projected
  line L8 (-7.8407, -59.4676) -> (-7.8323, -57.4676) projected
  arc A8 (-5.7137, -57.4166) -> (-7.8323, -57.4676) centre (-6.7723, -57.4721) ccw projected
  line L9 (-5.7137, -57.4166) -> (5.1968, -57.4628) projected
  arc A9 (7.3148, -57.5317) -> (5.1968, -57.4628) centre (6.2548, -57.5272) ccw projected
  line L10 (7.3148, -57.5317) -> (7.3064, -59.5317) projected
  arc A10 (5.1878, -59.5827) -> (7.3064, -59.5317) centre (6.2464, -59.5272) ccw projected
  line L11 (5.1878, -59.5827) -> (-5.7227, -59.5366) projected
  circle A11 centre (11.7442, -60.0505) radius 1.35 projected
  circle A12 centre (-0.1, -20) radius 4 projected
  line L12 (5.1861, -28.9475) -> (7.0991, -36.7384) projected
  arc A13 (5.7409, -39.1281) -> (7.0991, -36.7384) centre (5.1568, -37.2153) ccw projected
  arc A14 (-5.9409, -39.1281) -> (5.7409, -39.1281) centre (-0.1, -20) ccw projected
  arc A15 (-7.2991, -36.7384) -> (-5.9409, -39.1281) centre (-5.3568, -37.2153) ccw projected
  line L13 (-7.2991, -36.7384) -> (-5.3861, -28.9475) projected
  arc A16 (-2.775, -27.5395) -> (-5.3861, -28.9475) centre (-3.4438, -29.4244) ccw projected
  arc A17 (-2.775, -27.5395) -> (2.575, -27.5395) centre (-0.1, -20) ccw projected
  arc A18 (5.1861, -28.9475) -> (2.575, -27.5395) centre (3.2438, -29.4244) ccw projected
  line L14 (15.361, -62.5) -> (15.361, -54.5339) projected
  arc A19 (15.361, -54.5339) -> (15.2167, -53.3416) centre (10.361, -54.5339) ccw projected
  line L15 (15.2167, -53.3416) -> (6.62, -18.3308) projected
  arc A20 (6.62, -18.3308) -> (-6.9761, -18.3308) centre (-0.178, -20) ccw projected
  line L16 (-6.9761, -18.3308) -> (-15.5728, -53.3416) projected
  arc A21 (-15.5728, -53.3416) -> (-15.717, -54.5339) centre (-10.717, -54.5339) ccw projected
  line L17 (-15.717, -54.5339) -> (-15.717, -62.5) projected
  line L18 (-15.717, -62.5) -> (15.361, -62.5) projected
  line L19 (15.822, -61) -> (-16.178, -61)
  line L20 (-16.178, -61) -> (-16.178, -64)
  line L21 (-16.178, -64) -> (15.822, -64)
  line L22 (15.822, -64) -> (15.822, -61)
  line L23 (15.822, -61) -> (-16.178, -64) construction
  line L24 (-16.178, -61) -> (15.822, -64) construction
  line L25 (-16.178, -62.961) -> (-16.178, -54.5339)
  arc A22 (-16.0205, -53.2317) -> (-16.178, -54.5339) centre (-10.717, -54.5339) ccw
  line L26 (-16.0205, -53.2317) -> (-7.4238, -18.2208)
  arc A23 (7.0677, -18.2208) -> (-7.4238, -18.2208) centre (-0.178, -20) ccw
  line L27 (7.0677, -18.2208) -> (15.6644, -53.2317)
  arc A24 (15.822, -54.5339) -> (15.6644, -53.2317) centre (10.361, -54.5339) ccw
  line L28 (15.822, -54.5339) -> (15.822, -62.961)
  line L29 (15.822, -62.961) -> (-16.178, -62.961)
  point P0 (0, 0)
  point P1 (-0.178, -62.5)
  dimension "d93" = 32
  dimension "d94" = 3
  constraints: 22 end point, 6 point on circle, 3 centre point, 3 midpoint, 2 parallel, 1 horizontal, 1 perpendicular, 7 other
  measures "d93" distance of L21.end L20.end
  measures "d94" distance of L20.end L19.end
extrude "돌출24" add sketch "스케치24" against normal blind 2 contours L19 L25 A22 L26 A23 L27 A24 L28 L14 A19 L15 A20 L16 A21 L17 | L17 L18 L14 L19 L22 L29 L20
sketch "스케치25" plane through (0, 0, 2) normal (0, 0, 1) x (1, 0, 0)
  arc A0 (-15.6644, -53.2317) -> (-15.822, -54.5339) centre (-10.361, -54.5339) ccw projected
  line L0 (-15.822, -54.5339) -> (-15.822, -62.961) projected
  line L1 (-15.822, -62.961) -> (16.178, -62.961) projected
  line L2 (16.178, -62.961) -> (16.178, -54.5339) projected
  arc A1 (16.178, -54.5339) -> (16.0205, -53.2317) centre (10.717, -54.5339) ccw projected
  line L3 (16.0205, -53.2317) -> (7.4238, -18.2208) projected
  arc A2 (7.4238, -18.2208) -> (-7.0677, -18.2208) centre (0.178, -20) ccw projected
  line L4 (-7.0677, -18.2208) -> (-15.6644, -53.2317) projected
  circle A3 centre (-10.7928, -45.3463) radius 1.35 projected
  circle A4 centre (11.207, -45.2532) radius 1.35 projected
  arc A5 (6.1561, -47.3346) -> (8.2752, -47.3256) centre (7.2155, -47.2998) ccw projected
  line L5 (6.1561, -47.3346) -> (-5.7258, -47.3849) projected
  arc A6 (-7.8424, -47.3939) -> (-5.7258, -47.3849) centre (-6.7844, -47.3294) ccw projected
  line L6 (-7.8424, -47.3939) -> (-7.8441, -47.3939) projected
  line L7 (-7.8441, -47.3939) -> (-7.8616, -43.2739) projected
  line L8 (-7.8616, -43.2739) -> (-7.8599, -43.2739) projected
  arc A7 (-5.7433, -43.2649) -> (-7.8599, -43.2739) centre (-6.8013, -43.3294) ccw projected
  line L9 (-5.7433, -43.2649) -> (6.142, -43.2146) projected
  arc A8 (8.2544, -43.2057) -> (6.142, -43.2146) centre (7.1986, -43.2998) ccw projected
  line L10 (8.2544, -43.2057) -> (8.2583, -43.2057) projected
  line L11 (8.2583, -43.2057) -> (8.2757, -47.3256) projected
  line L12 (8.2757, -47.3256) -> (8.2752, -47.3256) projected
  circle A9 centre (12.2828, -59.9488) radius 1.35 projected
  arc A10 (5.7227, -59.5366) -> (7.8407, -59.4676) centre (6.7807, -59.4721) ccw projected
  line L13 (5.7227, -59.5366) -> (-5.1878, -59.5827) projected
  arc A11 (-7.3064, -59.5317) -> (-5.1878, -59.5827) centre (-6.2464, -59.5272) ccw projected
  line L14 (-7.3064, -59.5317) -> (-7.3148, -57.5317) projected
  arc A12 (-5.1968, -57.4628) -> (-7.3148, -57.5317) centre (-6.2548, -57.5272) ccw projected
  line L15 (-5.1968, -57.4628) -> (5.7137, -57.4166) projected
  arc A13 (7.8323, -57.4676) -> (5.7137, -57.4166) centre (6.7723, -57.4721) ccw projected
  line L16 (7.8323, -57.4676) -> (7.8407, -59.4676) projected
  circle A14 centre (-11.7442, -60.0505) radius 1.35 projected
  line L17 (-7.0991, -36.7384) -> (-5.1861, -28.9475) projected
  arc A15 (-2.575, -27.5395) -> (-5.1861, -28.9475) centre (-3.2438, -29.4244) ccw projected
  arc A16 (-2.575, -27.5395) -> (2.775, -27.5395) centre (0.1, -20) ccw projected
  arc A17 (5.3861, -28.9475) -> (2.775, -27.5395) centre (3.4438, -29.4244) ccw projected
  line L18 (5.3861, -28.9475) -> (7.2991, -36.7384) projected
  arc A18 (5.9409, -39.1281) -> (7.2991, -36.7384) centre (5.3568, -37.2153) ccw projected
  arc A19 (-5.7409, -39.1281) -> (5.9409, -39.1281) centre (0.1, -20) ccw projected
  arc A20 (-7.0991, -36.7384) -> (-5.7409, -39.1281) centre (-5.1568, -37.2153) ccw projected
  circle A21 centre (0.1, -20) radius 4 projected
  point P0 (0, 0)
extrude "돌출25" add sketch "스케치25" against normal blind 2 contours A3 | A4 | L5 A6 L7 A7 L9 A8 L10 L11 A5 | A9 | L13 A11 L14 A12 L15 A13 L16 A10 | A14 | L17 A15 A16 A17 L18 A18 A19 A20
sketch "스케치26" plane through (0, 0, 2) normal (0, 0, 1) x (1, 0, 0)
  arc A0 (-15.6644, -53.2317) -> (-15.822, -54.5339) centre (-10.361, -54.5339) ccw projected
  line L0 (-15.822, -54.5339) -> (-15.822, -62.961) projected
  line L1 (-15.822, -62.961) -> (16.178, -62.961) projected
  line L2 (16.178, -62.961) -> (16.178, -54.5339) projected
  arc A1 (16.178, -54.5339) -> (16.0205, -53.2317) centre (10.717, -54.5339) ccw projected
  line L3 (16.0205, -53.2317) -> (7.4238, -18.2208) projected
  arc A2 (7.4238, -18.2208) -> (-7.0677, -18.2208) centre (0.178, -20) ccw projected
  line L4 (-7.0677, -18.2208) -> (-15.6644, -53.2317) projected
  circle A3 centre (0.1, -20) radius 4 projected
  line L5 (-14.9, -62.961) -> (15.1, -62.961) projected
  line L6 (15.1, -62.961) -> (15.1, -54.5339) projected
  arc A4 (15.1, -54.5339) -> (14.9713, -53.4701) centre (10.639, -54.5339) ccw projected
  line L7 (14.9713, -53.4701) -> (6.3746, -18.4593) projected
  arc A5 (6.3746, -18.4593) -> (-6.1746, -18.4593) centre (0.1, -20) ccw projected
  line L8 (-6.1746, -18.4593) -> (-14.7713, -53.4701) projected
  arc A6 (-14.7713, -53.4701) -> (-14.9, -54.5339) centre (-10.439, -54.5339) ccw projected
  line L9 (-14.9, -54.5339) -> (-14.9, -62.961) projected
  line L10 (7.6736, -57.5) -> (7.6736, -59.5) projected
  arc A7 (5.5553, -59.56) -> (7.6736, -59.5) centre (6.6136, -59.5) ccw projected
  line L11 (5.5553, -59.56) -> (-5.3553, -59.56) projected
  arc A8 (-7.4736, -59.5) -> (-5.3553, -59.56) centre (-6.4136, -59.5) ccw projected
  line L12 (-7.4736, -59.5) -> (-7.4736, -57.5) projected
  arc A9 (-5.3553, -57.44) -> (-7.4736, -57.5) centre (-6.4136, -57.5) ccw projected
  line L13 (-5.3553, -57.44) -> (5.5553, -57.44) projected
  arc A10 (7.6736, -57.5) -> (5.5553, -57.44) centre (6.6136, -57.5) ccw projected
  circle A11 centre (-11.9136, -60) radius 1.35 projected
  circle A12 centre (12.1136, -60) radius 1.35 projected
  line L14 (-8.6217, -47.1327) -> (-4.5428, -30.5211) projected
  arc A13 (-0.3945, -27.4837) -> (-4.5428, -30.5211) centre (-0.6582, -31.475) ccw projected
  arc A14 (-0.3945, -27.4837) -> (0.5945, -27.4837) centre (0.1, -20) ccw projected
  arc A15 (4.7428, -30.5211) -> (0.5945, -27.4837) centre (0.8582, -31.475) ccw projected
  line L15 (4.7428, -30.5211) -> (8.8217, -47.1327) projected
  arc A16 (5.616, -52.0285) -> (8.8217, -47.1327) centre (4.9371, -48.0865) ccw projected
  arc A17 (-5.416, -52.0285) -> (5.616, -52.0285) centre (0.1, -20) ccw projected
  arc A18 (-8.6217, -47.1327) -> (-5.416, -52.0285) centre (-4.7371, -48.0865) ccw projected
  circle A19 centre (0.1, -20) radius 4 projected
  point P0 (0, 0)
extrude "돌출26" cut sketch "스케치26" against normal blind 2 contours L10 A7 L11 A8 L12 A9 L13 A10 | A11 | A12
sketch "스케치27" plane through (0, 0, 2) normal (0, 0, 1) x (1, 0, 0)
  circle A0 centre (-4.3, -45.3) radius 1 projected
  circle A1 centre (4.5, -45.3) radius 1 projected
  line L0 (8.1, -43.3) -> (8.1, -47.3) projected
  line L1 (-7.9, -43.3) -> (8.1, -43.3) projected
  line L2 (-7.9, -47.3) -> (-7.9, -43.3) projected
  line L3 (8.1, -47.3) -> (-7.9, -47.3) projected
  circle A2 centre (-10.9, -45.3) radius 1 projected
  circle A3 centre (11.1, -45.3) radius 1 projected
  circle A4 centre (11.1, -45.3) radius 1.35
  circle A5 centre (-10.9, -45.3) radius 1.35
  line L4 (-7.96, -47.36) -> (-7.96, -43.24)
  line L5 (-7.96, -43.24) -> (8.16, -43.24)
  line L6 (8.16, -43.24) -> (8.16, -47.36)
  line L7 (8.16, -47.36) -> (-7.96, -47.36)
  circle A6 centre (8.16, -47.36) radius 1.1
  circle A7 centre (8.16, -43.24) radius 1.1
  circle A8 centre (-7.96, -43.24) radius 1.1
  circle A9 centre (-7.96, -47.36) radius 1.1
  point P0 (0, 0)
  point P1 (-6.86, -47.36)
  point P2 (7.06, -47.36)
  point P3 (8.16, -46.26)
  point P4 (8.16, -44.34)
  point P5 (7.06, -43.24)
  point P6 (-6.86, -43.24)
  point P7 (-7.96, -44.34)
  point P8 (-7.96, -46.26)
  dimension "d101" = 2.7
  dimension "d102" = 2.7
  dimension "d107" = 0.06
  dimension "d109" = 2.2
  dimension "d110" = 2.2
  dimension "d111" = 2.2
  dimension "d112" = 2.2
  constraints: 8 end point, 6 centre point, 3 coincident, 3 other
  measures "d101" diameter of A4
  measures "d102" diameter of A5
  measures "d107" distance between parallel lines of L3 L7
  measures "d109" diameter of A6
  measures "d110" diameter of A7
  measures "d111" diameter of A8
  measures "d112" diameter of A9
extrude "돌출27" cut sketch "스케치27" against normal blind 2 contours A0 | A1 | L1 A7 L5 L6 L0 | L0 A7 L1 | A7 L6 A6 L0 | L0 A6 L3 A9 L2 A8 L1 A7 | L1 A8 L5 A7 | A6 L6 L7 L3 L0 | L0 L3 A6 | L6 L5 A7 | A8 L2 L1 | L1 L2 A8 L4 L5 | A6 L7 L6 | A6 L7 A9 L3 | L2 A9 L4 A8 | L5 L4 A8 | A9 L7 L4 L2 L3 | L3 L2 A9 | A9 L4 L7 | A2 | A3 | A4 | A5
sketch "스케치28" plane through (0, 0, 2) normal (0, 0, 1) x (1, 0, 0)
  line L0 (-14.9, -62.961) -> (15.1, -62.961) projected
  line L1 (15.1, -62.961) -> (15.1, -54.5339) projected
  arc A0 (15.1, -54.5339) -> (14.9713, -53.4701) centre (10.639, -54.5339) ccw projected
  line L2 (14.9713, -53.4701) -> (6.3746, -18.4593) projected
  arc A1 (6.3746, -18.4593) -> (-6.1746, -18.4593) centre (0.1, -20) ccw projected
  line L3 (-6.1746, -18.4593) -> (-14.7713, -53.4701) projected
  arc A2 (-14.7713, -53.4701) -> (-14.9, -54.5339) centre (-10.439, -54.5339) ccw projected
  line L4 (-14.9, -54.5339) -> (-14.9, -62.961) projected
  line L5 (7.6736, -57.5) -> (7.6736, -59.5) projected
  arc A3 (5.5553, -59.56) -> (7.6736, -59.5) centre (6.6136, -59.5) ccw projected
  line L6 (5.5553, -59.56) -> (-5.3553, -59.56) projected
  arc A4 (-7.4736, -59.5) -> (-5.3553, -59.56) centre (-6.4136, -59.5) ccw projected
  line L7 (-7.4736, -59.5) -> (-7.4736, -57.5) projected
  arc A5 (-5.3553, -57.44) -> (-7.4736, -57.5) centre (-6.4136, -57.5) ccw projected
  line L8 (-5.3553, -57.44) -> (5.5553, -57.44) projected
  arc A6 (7.6736, -57.5) -> (5.5553, -57.44) centre (6.6136, -57.5) ccw projected
  circle A7 centre (-11.9136, -60) radius 1.35 projected
  circle A8 centre (12.1136, -60) radius 1.35 projected
  line L9 (-8.6217, -47.1327) -> (-4.5428, -30.5211) projected
  arc A9 (-0.3945, -27.4837) -> (-4.5428, -30.5211) centre (-0.6582, -31.475) ccw projected
  arc A10 (-0.3945, -27.4837) -> (0.5945, -27.4837) centre (0.1, -20) ccw projected
  arc A11 (4.7428, -30.5211) -> (0.5945, -27.4837) centre (0.8582, -31.475) ccw projected
  line L10 (4.7428, -30.5211) -> (8.8217, -47.1327) projected
  arc A12 (5.616, -52.0285) -> (8.8217, -47.1327) centre (4.9371, -48.0865) ccw projected
  arc A13 (-5.416, -52.0285) -> (5.616, -52.0285) centre (0.1, -20) ccw projected
  arc A14 (-8.6217, -47.1327) -> (-5.416, -52.0285) centre (-4.7371, -48.0865) ccw projected
  circle A15 centre (0.1, -20) radius 4 projected
  line L11 (7.06, -43.24) -> (-6.86, -43.24) projected
  line L12 (0.1, -43.24) -> (0.1, -41.24)
  line L13 (0.1, -43.24) -> (2.1, -43.24) construction
  circle A16 centre (0.1, -20) radius 21.24
  point P0 (0, 0)
  point P1 (-6.8847, -40.0587)
  point P2 (7.0847, -40.0587)
  dimension "d115" = 2
  dimension "d116" = 90
  constraints: 4 end point, 2 perpendicular, 1 coincident, 1 horizontal, 1 midpoint, 3 other
  measures "d115" distance of L12.start L12.end
  measures "d116" angle of L13 L12
extrude "돌출28" cut sketch "스케치28" against normal blind 2 contours L9 A9 A10 A11 L10 A16
fillet "모깎기7" radius 2 2 edges at (7.0847, -40.0587, 1) (-6.8847, -40.0587, 1)
sketch "스케치29" plane through (0, 0, 2) normal (0, 0, 1) x (1, 0, 0)
  arc A0 (-4.9649, -40.6273) -> (5.1649, -40.6273) centre (0.1, -20) ccw projected
  arc A1 (-6.4303, -38.208) -> (-4.9649, -40.6273) centre (-4.488, -38.685) ccw projected
  line L0 (-6.4303, -38.208) -> (-4.5428, -30.5211) projected
  arc A2 (-0.3945, -27.4837) -> (-4.5428, -30.5211) centre (-0.6582, -31.475) ccw projected
  arc A3 (-0.3945, -27.4837) -> (0.5945, -27.4837) centre (0.1, -20) ccw projected
  arc A4 (4.7428, -30.5211) -> (0.5945, -27.4837) centre (0.8582, -31.475) ccw projected
  line L1 (4.7428, -30.5211) -> (6.6303, -38.208) projected
  arc A5 (5.1649, -40.6273) -> (6.6303, -38.208) centre (4.688, -38.685) ccw projected
  circle A6 centre (-10.9, -45.3) radius 1.35 projected
  line L2 (8.16, -44.34) -> (8.16, -46.26) projected
  arc A7 (7.06, -47.36) -> (8.16, -46.26) centre (8.16, -47.36) ccw projected
  line L3 (7.06, -47.36) -> (-6.86, -47.36) projected
  arc A8 (-7.96, -46.26) -> (-6.86, -47.36) centre (-7.96, -47.36) ccw projected
  line L4 (-7.96, -46.26) -> (-7.96, -44.34) projected
  arc A9 (-6.86, -43.24) -> (-7.96, -44.34) centre (-7.96, -43.24) ccw projected
  line L5 (-6.86, -43.24) -> (7.06, -43.24) projected
  arc A10 (8.16, -44.34) -> (7.06, -43.24) centre (8.16, -43.24) ccw projected
  circle A11 centre (11.1, -45.3) radius 1.35 projected
  circle A12 centre (-11.9136, -60) radius 1.35 projected
  arc A13 (-7.4736, -59.5) -> (-5.3553, -59.56) centre (-6.4136, -59.5) ccw projected
  line L6 (-7.4736, -59.5) -> (-7.4736, -57.5) projected
  arc A14 (-5.3553, -57.44) -> (-7.4736, -57.5) centre (-6.4136, -57.5) ccw projected
  line L7 (-5.3553, -57.44) -> (5.5553, -57.44) projected
  arc A15 (7.6736, -57.5) -> (5.5553, -57.44) centre (6.6136, -57.5) ccw projected
  line L8 (7.6736, -57.5) -> (7.6736, -59.5) projected
  arc A16 (5.5553, -59.56) -> (7.6736, -59.5) centre (6.6136, -59.5) ccw projected
  line L9 (5.5553, -59.56) -> (-5.3553, -59.56) projected
  circle A17 centre (12.1136, -60) radius 1.35 projected
  arc A18 (-15.6644, -53.2317) -> (-15.822, -54.5339) centre (-10.361, -54.5339) ccw projected
  line L10 (-15.822, -54.5339) -> (-15.822, -62.961) projected
  line L11 (-15.822, -62.961) -> (16.178, -62.961) projected
  line L12 (16.178, -62.961) -> (16.178, -54.5339) projected
  arc A19 (16.178, -54.5339) -> (16.0205, -53.2317) centre (10.717, -54.5339) ccw projected
  line L13 (16.0205, -53.2317) -> (7.4238, -18.2208) projected
  arc A20 (7.4238, -18.2208) -> (-7.0677, -18.2208) centre (0.178, -20) ccw projected
  line L14 (-7.0677, -18.2208) -> (-15.6644, -53.2317) projected
  circle A21 centre (0.1, -20) radius 4 projected
  line L15 (8.0492, -58) -> (16.178, -58)
  line L16 (16.178, -58) -> (16.178, -62)
  line L17 (16.178, -62) -> (8.0492, -62)
  line L18 (8.0492, -62) -> (8.0492, -58)
  line L19 (8.0492, -58) -> (16.178, -62) construction
  line L20 (16.178, -58) -> (8.0492, -62) construction
  line L21 (-8.0053, -58) -> (-15.822, -58)
  line L22 (-15.822, -58) -> (-15.822, -62)
  line L23 (-15.822, -62) -> (-8.0053, -62)
  line L24 (-8.0053, -62) -> (-8.0053, -58)
  line L25 (-8.0053, -58) -> (-15.822, -62) construction
  line L26 (-15.822, -58) -> (-8.0053, -62) construction
  line L27 (16.178, -62) -> (-15.822, -62)
  point P0 (0, 0)
  dimension "d120" = 4
  dimension "d121" = 4
  constraints: 26 end point, 4 midpoint, 4 parallel, 2 horizontal, 2 perpendicular, 2 point on line
  measures "d120" distance of L15.end L16.end
  measures "d121" distance of L22.end L21.end
extrude "돌출29" cut sketch "스케치29" against normal blind 2 contours L23 L27 L17 L12 L11 L10
sketch "스케치30" plane through (0, 0, 2) normal (0, 0, 1) x (1, 0, 0)
  circle A0 centre (0.1, -20) radius 4 projected
  line L0 (-15.822, -62) -> (16.178, -62) projected
  line L1 (16.178, -62) -> (16.178, -54.5339) projected
  arc A1 (16.178, -54.5339) -> (16.0205, -53.2317) centre (10.717, -54.5339) ccw projected
  line L2 (16.0205, -53.2317) -> (7.4238, -18.2208) projected
  arc A2 (7.4238, -18.2208) -> (-7.0677, -18.2208) centre (0.178, -20) ccw projected
  line L3 (-7.0677, -18.2208) -> (-15.6644, -53.2317) projected
  arc A3 (-15.6644, -53.2317) -> (-15.822, -54.5339) centre (-10.361, -54.5339) ccw projected
  line L4 (-15.822, -54.5339) -> (-15.822, -62) projected
  circle A4 centre (12.1136, -60) radius 1.35 projected
  arc A5 (-7.4736, -59.5) -> (-5.3553, -59.56) centre (-6.4136, -59.5) ccw projected
  line L5 (-7.4736, -59.5) -> (-7.4736, -57.5) projected
  arc A6 (-5.3553, -57.44) -> (-7.4736, -57.5) centre (-6.4136, -57.5) ccw projected
  line L6 (-5.3553, -57.44) -> (5.5553, -57.44) projected
  arc A7 (7.6736, -57.5) -> (5.5553, -57.44) centre (6.6136, -57.5) ccw projected
  line L7 (7.6736, -57.5) -> (7.6736, -59.5) projected
  arc A8 (5.5553, -59.56) -> (7.6736, -59.5) centre (6.6136, -59.5) ccw projected
  line L8 (5.5553, -59.56) -> (-5.3553, -59.56) projected
  circle A9 centre (-11.9136, -60) radius 1.35 projected
  circle A10 centre (11.1, -45.3) radius 1.35 projected
  line L9 (8.16, -44.34) -> (8.16, -46.26) projected
  arc A11 (7.06, -47.36) -> (8.16, -46.26) centre (8.16, -47.36) ccw projected
  line L10 (7.06, -47.36) -> (-6.86, -47.36) projected
  arc A12 (-7.96, -46.26) -> (-6.86, -47.36) centre (-7.96, -47.36) ccw projected
  line L11 (-7.96, -46.26) -> (-7.96, -44.34) projected
  arc A13 (-6.86, -43.24) -> (-7.96, -44.34) centre (-7.96, -43.24) ccw projected
  line L12 (-6.86, -43.24) -> (7.06, -43.24) projected
  arc A14 (8.16, -44.34) -> (7.06, -43.24) centre (8.16, -43.24) ccw projected
  circle A15 centre (-10.9, -45.3) radius 1.35 projected
  arc A16 (-4.9649, -40.6273) -> (5.1649, -40.6273) centre (0.1, -20) ccw projected
  arc A17 (-6.4303, -38.208) -> (-4.9649, -40.6273) centre (-4.488, -38.685) ccw projected
  line L13 (-6.4303, -38.208) -> (-4.5428, -30.5211) projected
  arc A18 (-0.3945, -27.4837) -> (-4.5428, -30.5211) centre (-0.6582, -31.475) ccw projected
  arc A19 (-0.3945, -27.4837) -> (0.5945, -27.4837) centre (0.1, -20) ccw projected
  arc A20 (4.7428, -30.5211) -> (0.5945, -27.4837) centre (0.8582, -31.475) ccw projected
  line L14 (4.7428, -30.5211) -> (6.6303, -38.208) projected
  arc A21 (5.1649, -40.6273) -> (6.6303, -38.208) centre (4.688, -38.685) ccw projected
  point P0 (0, 0)
extrude "돌출30" add sketch "스케치30" against normal blind 2 contours L5 A6 L6 A7 L7 A8 L8 A5
sketch "스케치32" plane through (0, 0, 2) normal (0, 0, 1) x (1, 0, 0)
  circle A0 centre (0.1, -20) radius 4 projected
  line L0 (-15.822, -62) -> (16.178, -62) projected
  line L1 (16.178, -62) -> (16.178, -54.5339) projected
  arc A1 (16.178, -54.5339) -> (16.0205, -53.2317) centre (10.717, -54.5339) ccw projected
  line L2 (16.0205, -53.2317) -> (7.4238, -18.2208) projected
  arc A2 (7.4238, -18.2208) -> (-7.0677, -18.2208) centre (0.178, -20) ccw projected
  line L3 (-7.0677, -18.2208) -> (-15.6644, -53.2317) projected
  arc A3 (-15.6644, -53.2317) -> (-15.822, -54.5339) centre (-10.361, -54.5339) ccw projected
  line L4 (-15.822, -54.5339) -> (-15.822, -62) projected
  circle A4 centre (12.1136, -60) radius 1.35 projected
  circle A5 centre (-11.9136, -60) radius 1.35 projected
  circle A6 centre (11.1, -45.3) radius 1.35 projected
  line L5 (8.16, -44.34) -> (8.16, -46.26) projected
  arc A7 (7.06, -47.36) -> (8.16, -46.26) centre (8.16, -47.36) ccw projected
  line L6 (7.06, -47.36) -> (-6.86, -47.36) projected
  arc A8 (-7.96, -46.26) -> (-6.86, -47.36) centre (-7.96, -47.36) ccw projected
  line L7 (-7.96, -46.26) -> (-7.96, -44.34) projected
  arc A9 (-6.86, -43.24) -> (-7.96, -44.34) centre (-7.96, -43.24) ccw projected
  line L8 (-6.86, -43.24) -> (7.06, -43.24) projected
  arc A10 (8.16, -44.34) -> (7.06, -43.24) centre (8.16, -43.24) ccw projected
  circle A11 centre (-10.9, -45.3) radius 1.35 projected
  arc A12 (-4.9649, -40.6273) -> (5.1649, -40.6273) centre (0.1, -20) ccw projected
  arc A13 (-6.4303, -38.208) -> (-4.9649, -40.6273) centre (-4.488, -38.685) ccw projected
  line L9 (-6.4303, -38.208) -> (-4.5428, -30.5211) projected
  arc A14 (-0.3945, -27.4837) -> (-4.5428, -30.5211) centre (-0.6582, -31.475) ccw projected
  arc A15 (-0.3945, -27.4837) -> (0.5945, -27.4837) centre (0.1, -20) ccw projected
  arc A16 (4.7428, -30.5211) -> (0.5945, -27.4837) centre (0.8582, -31.475) ccw projected
  line L10 (4.7428, -30.5211) -> (6.6303, -38.208) projected
  arc A17 (5.1649, -40.6273) -> (6.6303, -38.208) centre (4.688, -38.685) ccw projected
  point P0 (0, 0)
extrude "돌출32" add sketch "스케치32" against normal blind 2 contours A4 | A5